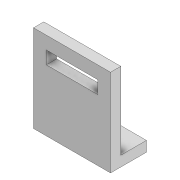
# Autodesk Inventor part: BatteryMount
Saved by Autodesk Inventor 2022 (Build 260153000, 153)
## iProperties
Created: 2022-10-26
Part Number: BatteryMount
Material: Generic
Document SubType Name: Modeling
Designer: MVeszpremi
Density: 1 g/cm^3
Appearance: Default
Author: MVeszpremi
Autodesk Inventor part; units mm, degrees
ref_plane "YZ Plane" through (0, 0, 0) normal (1, 0, 0) x (0, 1, 0)
ref_plane "XZ Plane" through (0, 0, 0) normal (0, 1, 0) x (-1, 0, 0)
ref_plane "XY Plane" through (0, 0, 0) normal (0, 0, 1) x (1, 0, 0)
sketch "Sketch1" plane through (0, 0, 0) normal (0, 1, 0) x (-1, 0, 0)
  line L0 (0, 0) -> (30, 0)
  line L1 (30, 0) -> (30, -10)
  line L2 (30, -10) -> (0, -10)
  line L3 (0, -10) -> (0, 0)
  circle A0 centre (22.5, -5) radius 1.5
  circle A1 centre (7.5, -5) radius 1.5
  dimension "d0" = 3
  dimension "d1" = 3
  dimension "d2" = 30
  dimension "d3" = 15
  dimension "d4" = 5
  dimension "d5" = 10
  dimension "d6" = 7.5
  constraints: 8 end point, 2 centre point, 2 parallel, 1 horizontal, 1 horizontal alignment, 1 perpendicular
  measures "d0" diameter of A0
  measures "d1" diameter of A1
  measures "d2" distance of L1.end L2.end
  measures "d3" distance of A1.centre A0.centre
  measures "d4" distance from line of L0 A0.centre
  measures "d5" distance of L0.end L1.end
  measures "d6" distance from line of L1 A0.centre
extrude "Extrusion1" add sketch "Sketch1" along normal blind 4
sketch "Sketch2" plane through (0, 4, 0) normal (0, 1, 0) x (1, 0, 0)
  line L0 (-30, 0) -> (0, 0) projected
  line L1 (0, 0) -> (-30, 0)
  line L2 (-30, 0) -> (-30, -4)
  line L3 (-30, -4) -> (0, -4)
  line L4 (0, -4) -> (0, 0)
  point P0 (-30, 0)
  dimension "d9" = 4
  constraints: 8 end point, 2 parallel, 1 horizontal, 1 perpendicular
  measures "d9" distance of L3.end L0.end
extrude "Extrusion2" add sketch "Sketch2" along normal blind 30 and the other way blind 4
sketch "Sketch3" plane through (-30, 34, 4) normal (0, 0, 1) x (1, 0, 0)
  line L0 (5, -5) -> (25, -5)
  line L1 (25, -5) -> (25, -10)
  line L2 (25, -10) -> (5, -10)
  line L3 (5, -10) -> (5, -5)
  line L4 (0, -34) -> (0, 0) projected
  line L5 (0, 0) -> (30, 0) projected
  point P0 (30, -34)
  dimension "d14" = 20
  dimension "d15" = 5
  dimension "d16" = 5
  dimension "d19" = 5
  constraints: 8 end point, 2 parallel, 1 horizontal, 1 perpendicular
  measures "d14" distance of L0.start L0.end
  measures "d15" distance between parallel lines of L4 L3
  measures "d16" distance between parallel lines of L0 L5
  measures "d19" distance of L0.end L1.end
extrude "Extrusion3" cut sketch "Sketch3" against normal blind 30
body "Solid1"
